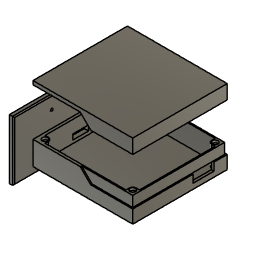
Case v15 (Autodesk Fusion 360 design; units mm, degrees)
part number: Configuration 1
Autodesk Fusion 360 part; units mm, degrees
sketch "Sketch1" plane through (0, 0, 0) normal (0, 0, 1) x (1, 0, 0) in component "Bottom"
  line L0 (0, 0) -> (190, 0)
  line L1 (190, 0) -> (190, 180)
  line L2 (190, 180) -> (0, 180)
  line L3 (0, 180) -> (0, 0)
  dimension "d1" = 190
  dimension "d2" = 180
  constraint horizontal L0
  constraint vertical L1
  constraint horizontal L2
  constraint vertical L3
  constraint coincident L0.start L3.end
  measures "d1" distance of L0.start L0.end
  measures "d2" distance of L0.start L2.end
extrude "Extrude1" add sketch "Sketch1" along normal blind 5 makes body 1 in component "Bottom"
sketch "Sketch2" plane through (0, 0, 5) normal (0, 0, 1) x (-1, 0, 0) in component "Bottom"
  line L0 (0, -180) -> (0, 0)
  line L1 (0, 0) -> (-190, 0)
  line L2 (-190, 0) -> (-190, -180)
  line L3 (-190, -180) -> (0, -180)
  line L4 (-5, -175) -> (-185, -175)
  line L5 (-185, -175) -> (-185, -5)
  line L6 (-185, -5) -> (-5, -5)
  line L7 (-5, -5) -> (-5, -175)
  circle A0 centre (-11.5, -168.5) radius 6.5
  circle A1 centre (-178.5, -168.5) radius 6.5
  circle A2 centre (-178.5, -11.5) radius 6.5
  circle A3 centre (-11.5, -11.5) radius 6.5
  line L8 (-11.5, -162) -> (-5, -162)
  line L9 (-18, -168.5) -> (-18, -175)
  line L10 (-172, -168.5) -> (-172, -175)
  line L11 (-178.5, -162) -> (-185, -162)
  line L12 (-178.5, -18) -> (-185, -18)
  line L13 (-172, -11.5) -> (-172, -5)
  line L14 (-18, -11.5) -> (-18, -5)
  line L15 (-5, -18) -> (-11.5, -18)
  dimension "d5" = 5
  dimension "d6" = 5
  dimension "d7" = 5
  dimension "d8" = 5
  dimension "d11" = 13
  constraint horizontal L4
  constraint vertical L5
  constraint horizontal L6
  constraint vertical L7
  constraint tangent L4 A0
  constraint tangent L7 A0
  constraint equal A0 A1
  constraint equal A0 A3
  constraint equal A0 A2
  constraint tangent L7 A3
  constraint tangent L6 A3
  constraint tangent L6 A2
  constraint tangent L5 A2
  constraint tangent L5 A1
  constraint tangent L4 A1
  constraint coincident A0 L8.start
  constraint coincident L7 L8.end
  constraint perpendicular L7 L8
  constraint tangent A0 L8
  constraint coincident A0 L9.start
  constraint coincident L4 L9.end
  constraint perpendicular L4 L9
  constraint coincident A1 L10.start
  constraint coincident L4 L10.end
  constraint perpendicular L4 L10
  constraint coincident A1 L11.start
  constraint coincident L5 L11.end
  constraint perpendicular L5 L11
  constraint coincident A2 L12.start
  constraint coincident L5 L12.end
  constraint perpendicular L5 L12
  constraint coincident A2 L13.start
  constraint coincident L6 L13.end
  constraint perpendicular L6 L13
  constraint coincident A3 L14.start
  constraint coincident L6 L14.end
  constraint perpendicular L6 L14
  constraint coincident L7 L15.start
  constraint coincident A3 L15.end
  constraint perpendicular L7 L15
  constraint tangent A3 L15
  constraint tangent A3 L14
  constraint tangent A2 L13
  constraint tangent A2 L12
  constraint tangent A1 L11
  constraint tangent A1 L10
  constraint tangent A0 L9
  measures "d5" horizontal distance of L0.start L4.start
  measures "d6" vertical distance of L0.start L4.start
  measures "d7" horizontal distance of L2.end L4.end
  measures "d8" vertical distance of L0.end L6.end
  measures "d11" diameter of A0
extrude "Extrude2" add sketch "Sketch2" along normal blind 40 contours L0 L1 L2 L3 | L4 A0 L9 | L4 A1 L10 | L4 L7 A0 | A0 | L4 L5 A1 | A1 | L7 A0 L8 | L5 A1 L11 | L7 A3 L15 | L5 A2 L12 | L6 L7 A3 | A3 | L5 L6 A2 | A2 | L6 A3 L14 | L6 A2 L13 bodies 1 in component "Bottom"
sketch "Sketch3" plane through (0, 0, 45) normal (0, 0, 1) x (-1, 0, 0) in component "Bottom"
  line L0 (-5, -162) -> (-11.5, -162)
  arc A0 (-11.5, -162) -> (-18, -168.5) centre (-11.5, -168.5) ccw
  line L1 (-18, -168.5) -> (-18, -175)
  line L2 (-18, -175) -> (-172, -175)
  line L3 (-172, -175) -> (-172, -168.5)
  arc A1 (-172, -168.5) -> (-178.5, -162) centre (-178.5, -168.5) ccw
  line L4 (-178.5, -162) -> (-185, -162)
  line L5 (-185, -162) -> (-185, -18)
  line L6 (-185, -18) -> (-178.5, -18)
  arc A2 (-178.5, -18) -> (-172, -11.5) centre (-178.5, -11.5) ccw
  line L7 (-172, -11.5) -> (-172, -5)
  line L8 (-172, -5) -> (-18, -5)
  line L9 (-18, -5) -> (-18, -11.5)
  arc A3 (-18, -11.5) -> (-11.5, -18) centre (-11.5, -11.5) ccw
  line L10 (-11.5, -18) -> (-5, -18)
  line L11 (-5, -18) -> (-5, -162)
  line L12 (-190, -180) -> (0, -180)
  line L13 (0, -180) -> (0, 0)
  line L14 (0, 0) -> (-190, 0)
  line L15 (-190, 0) -> (-190, -180)
  circle A4 centre (-11.5, -11.5) radius 5.5
  circle A5 centre (-178.5, -11.5) radius 5.5
  circle A6 centre (-178.5, -168.5) radius 5.5
  circle A7 centre (-11.5, -168.5) radius 5.5
  dimension "d12" = 11
  constraint concentric A3 A4
  constraint concentric A2 A5
  constraint concentric A1 A6
  constraint concentric A0 A7
  constraint equal A4 A7
  constraint equal A4 A5
  constraint equal A4 A6
  measures "d12" diameter of A4
extrude "Extrude3" cut sketch "Sketch3" against normal blind 4.6 contours A4 | A5 | A6 | A7 bodies 1 in component "Bottom"
sketch "Sketch4" plane through (0, 0, 45) normal (0, 0, 1) x (-1, 0, 0) in component "Bottom"
  line L0 (-185, -162) -> (-185, -18)
  line L1 (-185, -18) -> (-178.5, -18)
  arc A0 (-178.5, -18) -> (-172, -11.5) centre (-178.5, -11.5) ccw
  line L2 (-172, -11.5) -> (-172, -5)
  line L3 (-172, -5) -> (-18, -5)
  line L4 (-18, -5) -> (-18, -11.5)
  arc A1 (-18, -11.5) -> (-11.5, -18) centre (-11.5, -11.5) ccw
  line L5 (-11.5, -18) -> (-5, -18)
  line L6 (-5, -18) -> (-5, -162)
  line L7 (0, -180) -> (0, 0)
  line L8 (0, 0) -> (-190, 0)
  line L9 (-190, 0) -> (-190, -180)
  circle A2 centre (-11.5, -11.5) radius 5.5
  circle A3 centre (-178.5, -11.5) radius 5.5
  line L10 (-190, -180) -> (-90, -180)
  line L11 (-90, -180) -> (-90, -177.5)
  line L12 (-90, -177.5) -> (-190, -177.5)
  line L13 (-190, -177.5) -> (-190, -180)
  line L14 (-190, 0) -> (-90, 0)
  line L15 (-90, 0) -> (-90, -2.5)
  line L16 (-90, -2.5) -> (-190, -2.5)
  line L17 (-190, -2.5) -> (-190, 0)
  line L18 (-190, -177.5) -> (-190, -2.5)
  line L19 (-187.5, -177.5) -> (-187.5, -2.5)
  dimension "d39" = 100
  dimension "d40" = 2.5
  dimension "d41" = 100
  dimension "d42" = 2.5
  dimension "d43" = 2.5
  constraint horizontal L10
  constraint vertical L11
  constraint horizontal L12
  constraint vertical L13
  constraint coincident L9.end L10.start
  constraint horizontal L14
  constraint vertical L15
  constraint horizontal L16
  constraint vertical L17
  constraint coincident L8.end L9.start
  constraint coincident L12 L19.start
  constraint coincident L16 L19.end
  constraint perpendicular L16 L19
  measures "d39" distance of L9.end L10.end
  measures "d40" distance of L9.end L12.end
  measures "d41" distance of L8.end L14.end
  measures "d42" distance of L8.end L16.end
  measures "d43" distance of L18 L19
extrude "Extrude4" cut sketch "Sketch4" against normal blind 20 contours L8 L9 L14 L15 L16 L17 | L9 L12 L16 L18 L19 | L9 L10 L11 L12 L13 bodies 1 in component "Bottom"
chamfer "Chamfer1" distance 20 angle 45 2 edges at (90, 1.25, 25) (90, 178.75, 25) on bodies 1 in component "Bottom"
sketch "Sketch1 (2)" plane through (0, 180, 0) normal (0, 1, 0) x (-1, 0, 0)
  line L0 (-190, 25) -> (-190, 0)
  line L1 (-190, 0) -> (0, 0)
  line L2 (0, 0) -> (0, 45)
  line L3 (-85, 25) -> (-55, 25)
  line L4 (-55, 25) -> (-55, 10)
  line L5 (-55, 10) -> (-85, 10)
  line L6 (-85, 10) -> (-85, 25)
  line L7 (0, 45) -> (-90, 45)
  line L8 (-110, 25) -> (-190, 25)
  line L9 (-90, 45) -> (-110, 25)
  dimension "d21" = 30
  dimension "d22" = 15
  constraint horizontal L3
  constraint vertical L4
  constraint horizontal L5
  constraint vertical L6
  measures "d21" distance of L3.start L3.end
  measures "d22" distance of L3.start L5.end
sketch "Sketch1 (3)" plane through (0, 0, 45) normal (0, 0, 1) x (-1, 0, 0) in component "Top"
  line L0 (-5, -162) -> (-5, -18)
  line L1 (-5, -18) -> (-11.5, -18)
  arc A0 (-18, -11.5) -> (-11.5, -18) centre (-11.5, -11.5) ccw
  line L2 (-18, -11.5) -> (-18, -5)
  line L3 (-18, -5) -> (-172, -5)
  line L4 (-172, -5) -> (-172, -11.5)
  arc A1 (-178.5, -18) -> (-172, -11.5) centre (-178.5, -11.5) ccw
  line L5 (-178.5, -18) -> (-185, -18)
  line L6 (-185, -18) -> (-185, -162)
  line L7 (-185, -162) -> (-178.5, -162)
  arc A2 (-172, -168.5) -> (-178.5, -162) centre (-178.5, -168.5) ccw
  line L8 (-172, -168.5) -> (-172, -175)
  line L9 (-172, -175) -> (-18, -175)
  line L10 (-18, -175) -> (-18, -168.5)
  arc A3 (-11.5, -162) -> (-18, -168.5) centre (-11.5, -168.5) ccw
  line L11 (-11.5, -162) -> (-5, -162)
  line L12 (-90, 0) -> (-90, -2.5)
  line L13 (-90, -2.5) -> (-187.5, -2.5)
  line L14 (-187.5, -2.5) -> (-187.5, -177.5)
  line L15 (-187.5, -177.5) -> (-90, -177.5)
  line L16 (-90, -177.5) -> (-90, -180)
  line L17 (-90, -180) -> (0, -180)
  line L18 (0, -180) -> (0, 0)
  line L19 (0, 0) -> (-90, 0)
  line L20 (-5, -162) -> (-11.5, -162)
  arc A4 (-11.5, -162) -> (-18, -168.5) centre (-11.5, -168.5) ccw
  line L21 (-18, -168.5) -> (-18, -175)
  line L22 (-18, -175) -> (-172, -175)
  line L23 (-172, -175) -> (-172, -168.5)
  arc A5 (-172, -168.5) -> (-178.5, -162) centre (-178.5, -168.5) ccw
  line L24 (-178.5, -162) -> (-185, -162)
  line L25 (-185, -162) -> (-185, -18)
  line L26 (-185, -18) -> (-178.5, -18)
  arc A6 (-178.5, -18) -> (-172, -11.5) centre (-178.5, -11.5) ccw
  line L27 (-172, -11.5) -> (-172, -5)
  line L28 (-172, -5) -> (-18, -5)
  line L29 (-18, -5) -> (-18, -11.5)
  arc A7 (-18, -11.5) -> (-11.5, -18) centre (-11.5, -11.5) ccw
  line L30 (-11.5, -18) -> (-5, -18)
  line L31 (-5, -18) -> (-5, -162)
  circle A8 centre (-178.5, -168.5) radius 5.5
  circle A9 centre (-11.5, -168.5) radius 5.5
  circle A10 centre (-178.5, -11.5) radius 5.5
  circle A11 centre (-11.5, -11.5) radius 5.5
  line L32 (-110, -180) -> (-110, -177.5)
  line L33 (-110, -177.5) -> (-187.5, -177.5)
  line L34 (-187.5, -177.5) -> (-187.5, -2.5)
  line L35 (-187.5, -2.5) -> (-110, -2.5)
  line L36 (-110, -2.5) -> (-110, 0)
  line L37 (-110, 0) -> (-190, 0)
  line L38 (-190, 0) -> (-190, -180)
  line L39 (-190, -180) -> (-110, -180)
  line L40 (-90, -177.5) -> (-110, -177.5)
  line L41 (-110, -177.5) -> (-110, -180)
  line L42 (-110, -180) -> (-90, -180)
  line L43 (-90, -180) -> (-90, -177.5)
  line L44 (-90, 0) -> (-110, 0)
extrude "Extrude1'" add sketch "Sketch1 (3)" against normal blind 20 separate body contours L12 L13 L36 L44 | L13 L14 L15 L32 L33 L34 L35 L36 L37 L38 L39 L41 | L15 L16 L32 L40 L41 L42 L43 makes body 2 in component "Top"
chamfer "Chamfer1'" distance 20 angle 45 2 edges at (90, 178.75, 25) (90, 1.25, 25) on bodies 2 in component "Top"
sketch "Sketch2 (2)" plane through (0, 0, 45) normal (0, 0, 1) x (-1, 0, 0) in component "Top"
  line L0 (-90, 0) -> (-90, -2.5)
  line L1 (-90, -2.5) -> (-187.5, -2.5)
  line L2 (-187.5, -2.5) -> (-187.5, -177.5)
  line L3 (-187.5, -177.5) -> (-90, -177.5)
  line L4 (-90, -177.5) -> (-90, -180)
  line L5 (-90, -180) -> (0, -180)
  line L6 (0, -180) -> (0, 0)
  line L7 (0, 0) -> (-90, 0)
  line L8 (-5, -162) -> (-11.5, -162)
  arc A0 (-11.5, -162) -> (-18, -168.5) centre (-11.5, -168.5) ccw
  line L9 (-18, -168.5) -> (-18, -175)
  line L10 (-18, -175) -> (-172, -175)
  line L11 (-172, -175) -> (-172, -168.5)
  arc A1 (-172, -168.5) -> (-178.5, -162) centre (-178.5, -168.5) ccw
  line L12 (-178.5, -162) -> (-185, -162)
  line L13 (-185, -162) -> (-185, -18)
  line L14 (-185, -18) -> (-178.5, -18)
  arc A2 (-178.5, -18) -> (-172, -11.5) centre (-178.5, -11.5) ccw
  line L15 (-172, -11.5) -> (-172, -5)
  line L16 (-172, -5) -> (-18, -5)
  line L17 (-18, -5) -> (-18, -11.5)
  arc A3 (-18, -11.5) -> (-11.5, -18) centre (-11.5, -11.5) ccw
  line L18 (-11.5, -18) -> (-5, -18)
  line L19 (-5, -18) -> (-5, -162)
  circle A4 centre (-178.5, -168.5) radius 5.5
  circle A5 centre (-11.5, -168.5) radius 5.5
  circle A6 centre (-178.5, -11.5) radius 5.5
  circle A7 centre (-11.5, -11.5) radius 5.5
  line L20 (-90, -2.5) -> (-90, 0)
  line L21 (-90, 0) -> (-190, 0)
  line L22 (-190, 0) -> (-190, -180)
  line L23 (-190, -180) -> (-90, -180)
  line L24 (-90, -180) -> (-90, -177.5)
  line L25 (-90, -177.5) -> (-187.5, -177.5)
  line L26 (-187.5, -177.5) -> (-187.5, -2.5)
  line L27 (-187.5, -2.5) -> (-90, -2.5)
extrude "Extrude2'" add sketch "Sketch2 (2)" along normal blind 5 contours L0 L1 L2 L3 L4 L5 L6 L7 L20 L24 L25 L26 L27 | L0 L1 L2 L3 L4 L20 L21 L22 L23 L24 L25 L26 L27 | L8 A0 L9 L10 L11 A1 L12 L13 L14 A2 L15 L16 L17 A3 L18 L19 bodies 2 in component "Top"
sketch "Sketch3 (2)" plane through (0, 0, 50) normal (0, 0, 1) x (-1, 0, 0) in component "Top"
  circle A0 centre (-11.5, -11.5) radius 5.5
  circle A1 centre (-11.5, -168.5) radius 5.5
  circle A2 centre (-178.5, -11.5) radius 5.5
  circle A3 centre (-178.5, -168.5) radius 5.5
  line L0 (-190, -180) -> (0, -180)
  line L1 (0, -180) -> (0, 0)
  line L2 (0, 0) -> (-190, 0)
  line L3 (-190, 0) -> (-190, -180)
extrude "Extrude3'" add sketch "Sketch3 (2)" along normal blind 2 contours A0 | A1 | A2 | A3 | L0 L1 L2 L3 bodies 2 in component "Top"
sketch "Sketch6" plane through (190, 0, 0) normal (1, 0, 0) x (0, 1, 0) in component "Bottom"
  line L0 (180, 25) -> (0, 25)
  line L1 (0, 25) -> (0, 0)
  line L2 (0, 0) -> (180, 0)
  line L3 (180, 0) -> (180, 25)
  line L4 (115, 25) -> (155, 25)
  line L5 (155, 25) -> (155, 10)
  line L6 (155, 10) -> (115, 10)
  line L7 (115, 10) -> (115, 25)
  dimension "d44" = 40
  dimension "d45" = 15
  dimension "d46" = 25
  constraint horizontal L4
  constraint vertical L5
  constraint horizontal L6
  constraint vertical L7
  constraint coincident L0 L4.start
  measures "d44" distance of L4.start L4.end
  measures "d45" distance of L4.start L6.end
  measures "d46" horizontal distance of L2.end L5.end
extrude "Extrude6" cut sketch "Sketch6" against normal blind 35 contours L0 L4 L5 L6 L7 bodies 1 in component "Bottom"
sketch "Sketch7" plane through (0, 0, 0) normal (0, -1, 0) x (1, 0, 0) in component "Bottom"
  line L0 (90, 45) -> (0, 45)
  line L1 (0, 45) -> (0, 0)
  line L2 (0, 0) -> (190, 0)
  line L3 (190, 0) -> (190, 25)
  line L4 (190, 25) -> (110, 25)
  line L5 (110, 25) -> (90, 45)
  line L6 (31, 41) -> (30, 41)
  line L7 (0, 3) -> (0, 13)
  line L8 (45, 0) -> (45, 50)
  line L9 (11, 36) -> (15, 36)
  line L10 (30, 41) -> (30, 46)
  line L11 (15, 15) -> (15, 14)
  line L12 (0, 13) -> (26, 13)
  line L13 (26, 37) -> (0, 37)
  line L14 (28.5, 28) -> (29.5, 28)
  line L15 (0, 0) -> (45, 0)
  line L16 (45, 50) -> (0, 50)
  line L17 (29.5, 22) -> (28.5, 22)
  line L18 (11, 15) -> (15, 15)
  line L19 (0, 50) -> (0, 0)
  line L20 (0, 37) -> (0, 47)
  line L21 (26, 3) -> (0, 3)
  line L22 (30, 9) -> (31, 9)
  line L23 (31, 46) -> (31, 41)
  line L24 (15, 35) -> (11, 35)
  line L25 (11, 35) -> (11, 36)
  circle A0 centre (23, 25) radius 1.95
  line L26 (31, 4) -> (30, 4)
  line L27 (26, 13) -> (26, 3)
  line L28 (15, 14) -> (11, 14)
  line L29 (15, 36) -> (15, 35)
  line L30 (11, 14) -> (11, 15)
  line L31 (31, 9) -> (31, 4)
  line L32 (0, 47) -> (26, 47)
  line L33 (26, 47) -> (26, 37)
  line L34 (28.5, 22) -> (28.5, 28)
  line L35 (29.5, 28) -> (29.5, 22)
  line L36 (30, 4) -> (30, 9)
  line L37 (30, 46) -> (31, 46)
  point P0 (0, 25)
  point P1 (28.5, 25)
  dimension "d49" = 23
  dimension "d50" = 3.9
  dimension "d51" = 6
  dimension "d52" = 1
  dimension "d53" = 28.5
  dimension "d54" = 5
  dimension "d55" = 1
  dimension "d56" = 1
  dimension "d57" = 5
  dimension "d58" = 1
  dimension "d59" = 4
  dimension "d60" = 1
  dimension "d61" = 4
  dimension "d66" = 30
  dimension "d67" = 13
  dimension "d68" = 13
  dimension "d69" = 10
  dimension "d70" = 26
  dimension "d71" = 1
  dimension "d73" = 50
  dimension "d74" = 45
  dimension "d75" = 1
  dimension "d76" = 10
  dimension "d77" = 10
  dimension "d78" = 8
  dimension "d79" = 8
  constraint midpoint P0 L19
  constraint midpoint P1 L34
  constraint coincident L13.end L19
  constraint coincident L7.start L19
  constraint equal L7 L20
  constraint equal L13 L21
  constraint coincident L1.end L2.start
  constraint coincident L2 L8.start
  constraint coincident L0.end L19
  constraint perpendicular L8 L16
  constraint perpendicular L12 L27
  constraint perpendicular L21 L27
  constraint perpendicular L7 L12
  constraint coincident L7.end L19
  constraint perpendicular L9 L29
  constraint perpendicular L24 L29
  constraint perpendicular L24 L25
  constraint perpendicular L13 L33
  constraint perpendicular L32 L33
  constraint perpendicular L20 L32
  constraint coincident L20.end L19
  constraint perpendicular L11 L18
  constraint perpendicular L11 L28
  constraint perpendicular L28 L30
  constraint horizontal P0 A0.centre
  constraint equal L8 L19
  constraint perpendicular L6 L23
  constraint perpendicular L10 L37
  constraint perpendicular L23 L37
  constraint perpendicular L14 L35
  constraint perpendicular L17 L35
  constraint perpendicular L22 L31
  constraint perpendicular L26 L31
  constraint perpendicular L26 L36
  constraint vertical L6.end L22.start
  constraint horizontal A0.centre P1
  measures "d49" distance of A0.centre L19
  measures "d50" diameter of A0
  measures "d51" distance of L14.end L17.start
  measures "d52" distance of L14.start L14.end
  measures "d53" distance of L19 L34
  measures "d54" distance of L6.start L23.start
  measures "d55" distance of L23.start L10.end
  measures "d56" distance of L22.end L22.start
  measures "d57" distance of L26.start L22.end
  measures "d58" distance of L24.start L9.end
  measures "d59" distance of L9.start L9.end
  measures "d60" distance of L11.start L11.end
  measures "d61" distance of L11.start L18.start
  measures "d66" distance of L10 L19
  measures "d67" distance of L6 L14
  measures "d68" distance of L17 L22
  measures "d69" distance of L13.end L20.end
  measures "d70" distance of L13.end L13.start
  measures "d71" distance of L9 L13
  measures "d73" distance of L8.start L8.end
  measures "d74" distance of L8.start L1.end
  measures "d75" distance of L12 L28
  measures "d76" vertical distance of L24.start A0.centre
  measures "d77" vertical distance of L11.start A0.centre
  measures "d78" horizontal distance of L24.start A0.centre
  measures "d79" horizontal distance of L11.end A0.centre
extrude "Extrude7" [suppressed] in component "Bottom"
extrude "Extrude8" [suppressed] in component "Bottom"
sketch "Sketch8" plane through (0, 0, 0) normal (-1, 0, 0) x (0, -1, 0) in component "Bottom"
  line L0 (-180, 45) -> (-180, 0)
  line L1 (-180, 0) -> (0, 0)
  line L2 (0, 0) -> (0, 45)
  line L3 (0, 45) -> (-180, 45)
  line L4 (-220, 103.4) -> (40, 103.4)
  line L5 (40, 103.4) -> (40, -16.6)
  line L6 (40, -16.6) -> (-220, -16.6)
  line L7 (-220, -16.6) -> (-220, 103.4)
  point P0 (-90, -16.6)
  point P1 (-90, 0)
  dimension "d90" = 260
  dimension "d91" = 120
  dimension "d92" = 180
  dimension "d93" = 16.6
  constraint horizontal L4
  constraint vertical L5
  constraint horizontal L6
  constraint vertical L7
  constraint midpoint L6 P0
  constraint midpoint L1 P1
  constraint vertical P0 P1
  measures "d90" distance of L4.start L4.end
  measures "d91" distance of L4.start L6.end
  measures "d92" distance of L0.end L1.end
  measures "d93" distance of L1 L6
extrude "Extrude9" add sketch "Sketch8" along normal blind 8 contours L0 L1 L2 L3 | L4 L5 L6 L7 bodies 1 in component "Bottom"
sketch "Sketch9" plane through (-8, 0, 0) normal (-1, 0, 0) x (0, -1, 0) in component "Bottom"
  line L0 (-220, -16.6) -> (40, -16.6)
  line L1 (40, -16.6) -> (40, 103.4)
  line L2 (40, 103.4) -> (-220, 103.4)
  line L3 (-220, 103.4) -> (-220, -16.6)
  circle A0 centre (-35.8, 10.9) radius 1.5
  circle A1 centre (-135.8, 10.9) radius 1.5
  circle A2 centre (-35.8, 75.9) radius 1.5
  circle A3 centre (-135.8, 75.9) radius 1.5
  circle A4 centre (-35.8, 10.9) radius 3
  circle A5 centre (-135.8, 10.9) radius 3
  circle A6 centre (-35.8, 75.9) radius 3
  circle A7 centre (-135.8, 75.9) radius 3
  line L4 (-145.8, 99.4) -> (-25.8, 99.4)
  line L5 (-25.8, 99.4) -> (-25.8, 0.9)
  line L6 (-25.8, 0.9) -> (-145.8, 0.9)
  line L7 (-145.8, 0.9) -> (-145.8, 99.4)
  line L8 (-135.8, 72.9) -> (-145.8, 72.9)
  line L9 (-132.8, 75.9) -> (-132.8, 99.4)
  line L10 (-38.8, 75.9) -> (-38.8, 99.4)
  line L11 (-35.8, 72.9) -> (-25.8, 72.9)
  line L12 (-35.8, 13.9) -> (-25.8, 13.9)
  line L13 (-38.8, 10.9) -> (-38.8, 0.9)
  line L14 (-132.8, 10.9) -> (-132.8, 0.9)
  line L15 (-135.8, 13.9) -> (-145.8, 13.9)
  circle A8 centre (-35.8, 10.9) radius 2.5
  circle A9 centre (-135.8, 10.9) radius 2.5
  circle A10 centre (-35.8, 75.9) radius 2.5
  circle A11 centre (-135.8, 75.9) radius 2.5
  dimension "d96" = 3
  dimension "d99" = -100
  dimension "d100" = 65
  dimension "d101" = 27.5
  dimension "d103" = 120
  dimension "d106" = 6
  dimension "d110" = 10
  dimension "d111" = 10
  dimension "d113" = 10
  dimension "d116" = 5
  dimension "d117" = 4
  dimension "d134" = 75.8
  constraint concentric A0 A4
  constraint horizontal L4
  constraint vertical L5
  constraint horizontal L6
  constraint vertical L7
  constraint coincident A7 L8.start
  constraint coincident L7 L8.end
  constraint perpendicular L7 L8
  constraint coincident A7 L9.start
  constraint coincident L4 L9.end
  constraint perpendicular L4 L9
  constraint tangent A7 L9
  constraint tangent A7 L8
  constraint coincident A6 L10.start
  constraint coincident L4 L10.end
  constraint tangent A6 L10
  constraint perpendicular L4 L10
  constraint coincident A6 L11.start
  constraint coincident L5 L11.end
  constraint tangent A6 L11
  constraint perpendicular L5 L11
  constraint coincident A4 L12.start
  constraint coincident L5 L12.end
  constraint tangent A4 L12
  constraint coincident A4 L13.start
  constraint coincident L6 L13.end
  constraint perpendicular L12 L13
  constraint perpendicular L6 L13
  constraint tangent A4 L13
  constraint coincident A5 L14.start
  constraint coincident L6 L14.end
  constraint perpendicular L6 L14
  constraint coincident A5 L15.start
  constraint coincident L7 L15.end
  constraint perpendicular L7 L15
  constraint tangent A5 L15
  constraint tangent A5 L14
  constraint concentric A0 A8
  measures "d96" diameter of A0
  measures "d101" vertical distance of L0.end A0.centre
  measures "d103" distance of L0.end L1.end
  measures "d106" diameter of A4
  measures "d110" horizontal distance of A0.centre L5.end
  measures "d111" vertical distance of A0.centre L5.end
  measures "d113" horizontal distance of A3.centre L4.start
  measures "d116" diameter of A8
  measures "d117" vertical distance of L2.end L4.start
  measures "d134" horizontal distance of L0.end A0.centre
extrude "Extrude10" cut sketch "Sketch9" against normal blind 25 contours A0 | A1 | A2 | A3 bodies 1 in component "Bottom"
extrude "Extrude11" cut sketch "Sketch9" against normal blind 15 from surface at -2 contours A8 | A9 | A10 | A11 bodies 1 in component "Bottom"
extrude "Extrude12" cut sketch "Sketch9" against normal blind 5 contours A4 A5 A6 A7 L4 L5 L6 L7 L8 L9 L10 L11 L12 L13 L14 L15 bodies 1 in component "Bottom"
sketch "Sketch10" plane through (-8, 0, 0) normal (-1, 0, 0) x (0, -1, 0) in component "Bottom"
  line L0 (-38.8, 0.9) -> (-132.8, 0.9)
  line L1 (-132.8, 0.9) -> (-132.8, 10.9)
  arc A0 (-132.8, 10.9) -> (-135.8, 13.9) centre (-135.8, 10.9) ccw
  line L2 (-135.8, 13.9) -> (-145.8, 13.9)
  line L3 (-145.8, 13.9) -> (-145.8, 72.9)
  line L4 (-145.8, 72.9) -> (-135.8, 72.9)
  arc A1 (-135.8, 72.9) -> (-132.8, 75.9) centre (-135.8, 75.9) ccw
  line L5 (-132.8, 75.9) -> (-132.8, 99.4)
  line L6 (-132.8, 99.4) -> (-38.8, 99.4)
  line L7 (-38.8, 99.4) -> (-38.8, 75.9)
  arc A2 (-38.8, 75.9) -> (-35.8, 72.9) centre (-35.8, 75.9) ccw
  line L8 (-35.8, 72.9) -> (-25.8, 72.9)
  line L9 (-25.8, 72.9) -> (-25.8, 13.9)
  line L10 (-25.8, 13.9) -> (-35.8, 13.9)
  arc A3 (-35.8, 13.9) -> (-38.8, 10.9) centre (-35.8, 10.9) ccw
  line L11 (-38.8, 10.9) -> (-38.8, 0.9)
  circle A4 centre (-135.8, 10.9) radius 1.5
  circle A5 centre (-35.8, 10.9) radius 1.5
  circle A6 centre (-135.8, 75.9) radius 1.5
  circle A7 centre (-35.8, 75.9) radius 1.5
  line L12 (-220, -16.6) -> (40, -16.6)
  line L13 (40, -16.6) -> (40, 103.4)
  line L14 (40, 103.4) -> (-220, 103.4)
  line L15 (-220, 103.4) -> (-220, -16.6)
  line L16 (-218, 101.4) -> (-218, -14.6)
  line L17 (-218, -14.6) -> (38, -14.6)
  line L18 (38, -14.6) -> (38, 101.4)
  line L19 (38, 101.4) -> (-218, 101.4)
  dimension "d118" = -2
extrude "Extrude13" add sketch "Sketch10" along normal blind 11 contours L12 L13 L14 L15 bodies 1 in component "Bottom"
sketch "Sketch11" plane through (-3, 0, 0) normal (-1, 0, 0) x (0, -1, 0) in component "Bottom"
  line L0 (-132.8, 10.9) -> (-132.8, 0.9)
  line L1 (-132.8, 0.9) -> (-38.8, 0.9)
  line L2 (-38.8, 0.9) -> (-38.8, 10.9)
  arc A0 (-35.8, 13.9) -> (-38.8, 10.9) centre (-35.8, 10.9) ccw
  line L3 (-35.8, 13.9) -> (-25.8, 13.9)
  line L4 (-25.8, 13.9) -> (-25.8, 72.9)
  line L5 (-25.8, 72.9) -> (-35.8, 72.9)
  arc A1 (-38.8, 75.9) -> (-35.8, 72.9) centre (-35.8, 75.9) ccw
  line L6 (-38.8, 75.9) -> (-38.8, 99.4)
  line L7 (-38.8, 99.4) -> (-132.8, 99.4)
  line L8 (-132.8, 99.4) -> (-132.8, 75.9)
  arc A2 (-135.8, 72.9) -> (-132.8, 75.9) centre (-135.8, 75.9) ccw
  line L9 (-135.8, 72.9) -> (-145.8, 72.9)
  line L10 (-145.8, 72.9) -> (-145.8, 13.9)
  line L11 (-145.8, 13.9) -> (-135.8, 13.9)
  arc A3 (-132.8, 10.9) -> (-135.8, 13.9) centre (-135.8, 10.9) ccw
  line L12 (-100.8, 10.9) -> (-70.8, 10.9)
  line L13 (-70.8, 10.9) -> (-70.8, 20.9)
  line L14 (-70.8, 20.9) -> (-100.8, 20.9)
  line L15 (-100.8, 20.9) -> (-100.8, 10.9)
  point P0 (-85.8, 10.9)
  point P1 (-85.8, 0.9)
  dimension "d121" = 10
  dimension "d122" = 30
  constraint horizontal L12
  constraint vertical L13
  constraint horizontal L14
  constraint vertical L15
  constraint horizontal A3.centre L12.start
  constraint midpoint L12 P0
  constraint midpoint L1 P1
  constraint vertical P0 P1
  measures "d121" distance of L12.end L13.end
  measures "d122" distance of L13.end L14.end
extrude "Extrude14" cut sketch "Sketch11" against normal blind 10 contours L12 L13 L14 L15 bodies 1 in component "Bottom"
fillet "Fillet1" radius 2.5 4 edges at (-9.5, 220, 103.4) (-9.5, 220, -16.6) (-9.5, -40, -16.6) (-9.5, -40, 103.4) on bodies 1 in component "Bottom"
chamfer "Chamfer3" distance 1 angle 45 8 edges at (0, 90, 103.4) (0, -39.2678, 102.6678) (0, -40, 43.4) (0, -39.2678, -15.8678) (0, 90, -16.6) (0, 219.2678, -15.8678) (0, 220, 43.4) (0, 219.2678, 102.6678) on bodies 1 in component "Bottom"
sketch "Sketch12" plane through (-19, 0, 0) normal (-1, 0, 0) x (0, -1, 0) in component "Bottom"
  arc A0 (40, 100.9) -> (37.5, 103.4) centre (37.5, 100.9) ccw
  line L0 (37.5, 103.4) -> (-217.5, 103.4)
  arc A1 (-217.5, 103.4) -> (-220, 100.9) centre (-217.5, 100.9) ccw
  line L1 (-220, 100.9) -> (-220, -14.1)
  arc A2 (-220, -14.1) -> (-217.5, -16.6) centre (-217.5, -14.1) ccw
  line L2 (-217.5, -16.6) -> (37.5, -16.6)
  arc A3 (37.5, -16.6) -> (40, -14.1) centre (37.5, -14.1) ccw
  line L3 (40, -14.1) -> (40, 100.9)
  line L4 (-218, 101.4) -> (38, 101.4)
  line L5 (38, 101.4) -> (38, -14.6)
  line L6 (38, -14.6) -> (-218, -14.6)
  line L7 (-218, -14.6) -> (-218, 101.4)
  line L8 (40, -16.6) -> (-220, -16.6)
  line L9 (-220, -16.6) -> (-220, 103.4)
  line L10 (-220, 103.4) -> (40, 103.4)
  line L11 (40, 103.4) -> (40, -16.6)
  line L12 (37, -13.6) -> (-217, -13.6)
  line L13 (-217, -13.6) -> (-217, 100.4)
  line L14 (-217, 100.4) -> (37, 100.4)
  line L15 (37, 100.4) -> (37, -13.6)
  dimension "d129" = 3
  constraint horizontal L8
  constraint vertical L9
  constraint horizontal L10
  constraint vertical L11
  constraint horizontal L0.end L9.end
  constraint vertical A1.end L9.end
  constraint vertical A3.end L8.start
  constraint horizontal L2.end L8.start
extrude "Extrude15" cut sketch "Sketch12" against normal blind 30 contours A0 L0 A1 L1 A2 L2 A3 L3 L8 L9 L10 L11 | L4 L5 L6 L7 bodies 1 in component "Bottom"
chamfer "Chamfer4" distance 2 angle 45 4 edges at (0, 90, 100.4) (0, -37, 43.4) (0, 90, -13.6) (0, 217, 43.4) on bodies 1 in component "Bottom"
component "Bottom" placed x (1, 0, 0) y (0, 1, 0) z (0, 0, 1) at (0, 0, 0)
component "Top" placed x (1, 0, 0) y (0, 1, 0) z (0, 0, 1) at (0, 0, 0)
equation "d6 = d5"
equation "d7 = d5"
equation "d8 = d5"
equation "d77 = d76"
equation "d79 = d78"
equation "d93 = 23.6 mm + 8 mm - 5 mm - 10 mm"
equation "d101 = ( d103 - 65 mm ) / 2"
equation "d111 = d110"
equation "d113 = d110"
equation "d134 = 71.8 mm + 4 mm"
